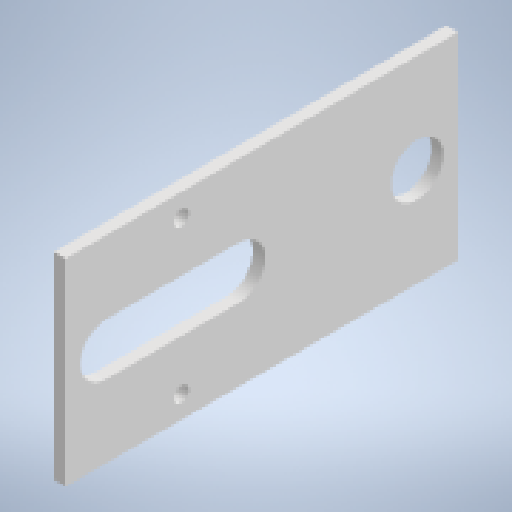
# Autodesk Inventor part: motorPlate
Saved by Autodesk Inventor 2023 (Build 270158000, 158)
## iProperties
Created: 2022-09-25
Part Number: motorPlate
Material: Generic
Document SubType Name: Modeling
Designer: deli
Density: 1 g/cm^3
Appearance: Default
Author: deli
Autodesk Inventor part; units mm, degrees
ref_plane "YZ Plane" through (0, 0, 0) normal (1, 0, 0) x (0, 1, 0)
ref_plane "XZ Plane" through (0, 0, 0) normal (0, 1, 0) x (-1, 0, 0)
ref_plane "XY Plane" through (0, 0, 0) normal (0, 0, 1) x (1, 0, 0)
sketch "Sketch1" plane through (0, 0, 0) normal (1, 0, 0) x (0, 1, 0)
  line L0 (42.0428, 1.6766) -> (-10.9572, 1.6766)
  line L1 (-10.9572, 1.6766) -> (-10.9572, -103.6949)
  line L2 (-10.9572, -103.6949) -> (42.0428, -103.6949)
  line L3 (42.0428, -103.6949) -> (42.0428, 1.6766)
  circle A0 centre (15.5428, -92.6949) radius 7
  arc A1 (22.5428, -9.3234) -> (8.5428, -9.3234) centre (15.5428, -9.3234) ccw
  circle A2 centre (15.5428, -9.3234) radius 13.5 construction
  circle A3 centre (36.0428, -29.3234) radius 5 construction
  line L4 (40.4393, -26.942) -> (27.4133, -2.8937) construction
  circle A4 centre (-4.9572, -29.3234) radius 5 construction
  line L5 (3.6724, -2.8937) -> (-9.3536, -26.942) construction
  circle A5 centre (15.5428, -92.6949) radius 13.5 construction
  line L6 (40.9576, -30.2427) -> (28.8127, -95.1768) construction
  line L7 (2.273, -95.1768) -> (-9.8719, -30.2427) construction
  arc A6 (8.5428, -44.8234) -> (22.5428, -44.8234) centre (15.5428, -44.8234) ccw
  line L8 (22.5428, -9.3234) -> (22.5428, -44.8234)
  line L9 (8.5428, -44.8234) -> (8.5428, -9.3234)
  circle A7 centre (15.5428, -44.8234) radius 13.5 construction
  circle A8 centre (36.0428, -29.3234) radius 2
  circle A9 centre (-4.9572, -29.3234) radius 2
  circle A10 centre (15.5428, -71.3234) radius 7
  circle A11 centre (15.5428, -44.8234) radius 18.5 construction
  point P0 (0, 0)
  dimension "d0" = 53
  dimension "d1" = 14
  dimension "d2" = 26.5
  dimension "d3" = 14
  dimension "d4" = 26.5
  dimension "d5" = 4
  dimension "d6" = 27
  dimension "d7" = 10
  dimension "d8" = 20.5
  dimension "d9" = 10
  dimension "d10" = 20.5
  dimension "d11" = 123.115
  dimension "d14" = 20
  dimension "d15" = 20
  dimension "d16" = 27
  dimension "d17" = 66.0602
  dimension "d18" = 27.3496
  dimension "d19" = 39.036
  dimension "d20" = 158.812
  dimension "d22" = 14
  dimension "d23" = 27
  dimension "d24" = 15.5
  dimension "d25" = 6
  dimension "d26" = 4
  dimension "d27" = 4
  dimension "d28" = 4
  dimension "d31" = 14
  dimension "d32" = 26.5
  dimension "d34" = 5
  dimension "d35" = 1
  constraints: 20 end point, 12 centre point, 12 point on circle, 12 tangent, 6 coincident, 2 parallel, 1 horizontal, 1 perpendicular, 1 vertical
  measures "d0" distance of L0.start L0.end
  measures "d1" diameter of A0
  measures "d2" distance from line of L3 A0.centre
  measures "d3" diameter of A1
  measures "d4" distance from line of L3 A1.centre
  measures "d5" distance edge to line of A1 L0
  measures "d6" diameter of A2
  measures "d7" diameter of A3
  measures "d8" horizontal distance of A3.centre A1.centre
  measures "d9" diameter of A4
  measures "d10" horizontal distance of A4.centre A1.centre
  measures "d14" vertical distance of A3.centre A1.centre
  measures "d15" vertical distance of A4.centre A1.centre
  measures "d16" diameter of A5
  measures "d17" distance of L6.start L6.end
  measures "d18" distance of L4.start L4.end
  measures "d22" diameter of A6
  measures "d23" diameter of A7
  measures "d24" vertical distance of A6.centre A3.centre
  measures "d25" distance from line of A3.centre L3
  measures "d26" diameter of A8
  measures "d27" diameter of A9
  measures "d28" distance edge to line of A0 L2
  measures "d31" diameter of A10
  measures "d32" distance from line of L3 A10.centre
  measures "d34" radial gap between concentric circles of A11 A7
extrude "Extrusion1" add sketch "Sketch1" along normal blind 3.175
equation "\"d2\" = 0.5 * d0"
equation "\"d3\" = d1"
equation "\"d4\" = d2"
equation "\"d9\" = d7"
equation "\"d10\" = d8"
equation "\"d15\" = d14"
equation "\"d16\" = d6"
equation "\"d22\" = d3"
equation "\"d23\" = d6"
equation "\"d27\" = d26"
equation "\"d31\" = d1"
equation "\"d32\" = d4"
body "Solid1"
